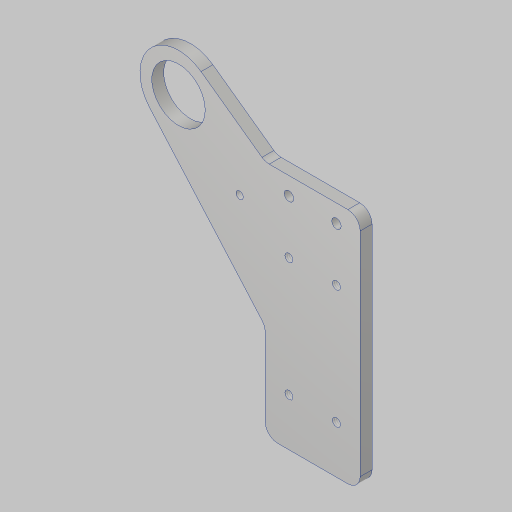
# Autodesk Inventor part: CL7-GB-008
Saved by Autodesk Inventor 2023.5 (Build 275446000, 446)
## iProperties
Created: 2025-03-18
Part Number: CL7-GB-008
Material: Aluminum 6061
Document SubType Name: Modeling
Designer: slick
Density: 2.7 g/cm^3
Appearance: Aluminum - Flat
Mass: 158.098 g
Surface Area: 311.728 cm^2
Volume: 58.555 cm^3
Author: slick
Autodesk Inventor part; units mm, degrees
ref_plane "YZ Plane" through (0, 0, 0) normal (1, 0, 0) x (0, 1, 0)
ref_plane "XZ Plane" through (0, 0, 0) normal (0, 1, 0) x (-1, 0, 0)
ref_plane "XY Plane" through (0, 0, 0) normal (0, 0, 1) x (1, 0, 0)
sketch "Sketch1" plane through (0, 0, 0) normal (0, 0, 1) x (1, 0, 0)
  line L0 (0, 0) -> (-50.8, 0) construction
  line L1 (-50.8, 0) -> (-50.8, 381) construction
  line L2 (-50.8, 381) -> (0, 381) construction
  line L3 (0, 381) -> (0, 0) construction
  circle A0 centre (-50.8, 431.8) radius 11.1125 construction
  line L4 (-50.8, 353.7099) -> (-298.4703, 0) construction
  line L5 (-298.4703, 0) -> (-267.4626, 0) construction
  line L6 (-267.4626, 0) -> (-50.8, 309.4263) construction
  dimension "d0" = 50.8
  dimension "d1" = 381
  dimension "d2" = 22.225
  dimension "d3" = 431.8
  dimension "d4" = 50.8
  dimension "d5" = 431.8
  dimension "d6" = 25.4
  dimension "d7" = 35
  constraints: 14 end point, 3 parallel, 2 horizontal, 2 point on line, 1 centre point, 1 collinear, 1 perpendicular
  measures "d0" distance of L1.end L2.end
  measures "d1" distance of L0.end L1.end
  measures "d2" diameter of A0
  measures "d3" distance from line of L0 A0.centre
  measures "d4" distance from line of L3 A0.centre
  measures "d5" distance of L4.start L4.end
  measures "d6" distance between parallel lines of L6 L4
  measures "d7" angle of L1 L4
sketch "Sketch2" plane through (0, 0, 0) normal (0, 0, 1) x (1, 0, 0)
  line L0 (-267.4626, 0) -> (-50.8, 309.4263) construction
  line L1 (-50.8, 353.7099) -> (-298.4703, 0) construction
  line L2 (-50.8, 0) -> (-50.8, 381) construction
  line L3 (0, 381) -> (0, 0) construction
  line L4 (-50.8, 381) -> (0, 381) construction
  circle A0 centre (-50.8, 431.8) radius 11.1125 construction
  line L5 (0, 0) -> (-50.8, 0) construction
  line L6 (-298.4703, 0) -> (-267.4626, 0) construction
  circle A1 centre (-88.9, 38.1) radius 30.48 construction
  circle A2 centre (-88.9, 38.1) radius 6.35 construction
  circle A3 centre (-124.3919, 76.2) radius 45.72 construction
  circle A4 centre (-124.3919, 76.2) radius 11.43 construction
  circle A5 centre (-101.6, 129.9906) radius 46.99 construction
  circle A6 centre (-101.6, 129.9906) radius 12.7 construction
  circle A7 centre (-97.155, 185.6935) radius 43.18 construction
  circle A8 centre (-124.3919, 76.2) radius 14.2875
  circle A9 centre (-101.6, 129.9906) radius 14.2875
  circle A10 centre (-97.155, 185.6935) radius 14.2875
  circle A11 centre (-50.8, 431.8) radius 54.5719 construction
  line L7 (-50.8, 177.8) -> (0, 177.8)
  circle A12 centre (-97.155, 185.6935) radius 20.6375 construction
  circle A13 centre (-101.6, 129.9906) radius 20.6375 construction
  circle A14 centre (-124.3919, 76.2) radius 20.6375 construction
  circle A15 centre (-88.9, 38.1) radius 25.4 construction
  line L8 (-50.8, 177.8) -> (-85.1131, 202.4536)
  line L9 (-141.8793, 65.2411) -> (-114.7275, 21.9145)
  line L10 (-74.6041, 11.1805) -> (0, 50.8)
  line L11 (0, 177.8) -> (0, 50.8)
  arc A16 (-141.8226, 87.2489) -> (-117.7308, 184.0988) centre (-275.3417, 171.8837) ccw
  arc A17 (-85.1131, 202.4536) -> (-117.7308, 184.0988) centre (-97.155, 185.6935) ccw
  arc A18 (-141.8226, 87.2489) -> (-141.8793, 65.2411) centre (-124.3919, 76.2) ccw
  arc A19 (-114.7275, 21.9145) -> (-74.6041, 11.1805) centre (-88.9, 38.1) ccw
  line L12 (-38.1, 152.4) -> (-38.1, 127) construction
  line L13 (-40.6527, 152.4) -> (-40.6527, 127)
  line L14 (-35.5473, 127) -> (-35.5473, 152.4)
  arc A20 (-35.5473, 152.4) -> (-40.6527, 152.4) centre (-38.1, 152.4) ccw
  arc A21 (-40.6527, 127) -> (-35.5473, 127) centre (-38.1, 127) ccw
  line L15 (-12.7, 152.4) -> (-12.7, 127) construction
  line L16 (-15.2527, 152.4) -> (-15.2527, 127)
  line L17 (-10.1473, 127) -> (-10.1473, 152.4)
  arc A22 (-10.1473, 152.4) -> (-15.2527, 152.4) centre (-12.7, 152.4) ccw
  arc A23 (-15.2527, 127) -> (-10.1473, 127) centre (-12.7, 127) ccw
  line L18 (-38.1, 139.7) -> (-12.7, 139.7) construction
  line L19 (-38.1, 88.9) -> (-38.1, 63.5) construction
  line L20 (-40.6527, 88.9) -> (-40.6527, 63.5)
  line L21 (-35.5473, 63.5) -> (-35.5473, 88.9)
  arc A24 (-35.5473, 88.9) -> (-40.6527, 88.9) centre (-38.1, 88.9) ccw
  arc A25 (-40.6527, 63.5) -> (-35.5473, 63.5) centre (-38.1, 63.5) ccw
  line L22 (-12.7, 88.9) -> (-12.7, 63.5) construction
  line L23 (-15.2527, 88.9) -> (-15.2527, 63.5)
  line L24 (-10.1473, 63.5) -> (-10.1473, 88.9)
  arc A26 (-10.1473, 88.9) -> (-15.2527, 88.9) centre (-12.7, 88.9) ccw
  arc A27 (-15.2527, 63.5) -> (-10.1473, 63.5) centre (-12.7, 63.5) ccw
  line L25 (-38.1, 76.2) -> (-12.7, 76.2) construction
  circle A28 centre (-88.9, 38.1) radius 10.795
  line L26 (-112.6649, 172.0793) -> (-50.8, 101.6)
  line L27 (-50.8, 101.6) -> (-50.8, 23.822)
  arc A29 (-117.7308, 184.0988) -> (-112.6649, 172.0793) centre (-97.155, 185.6935) ccw
  line L28 (0, 50.8) -> (-50.8, 50.8)
  point P0 (-88.9, 63.5)
  point P1 (-110.897, 50.8)
  point P2 (-110.897, 25.4)
  point P3 (-88.9, 12.7)
  point P4 (-66.903, 25.4)
  point P5 (-66.903, 50.8)
  point P6 (-25.4, 139.7)
  point P7 (-25.4, 177.8)
  point P8 (-25.4, 76.2)
  point P9 (-38.1, 168.275)
  point P10 (-12.7, 168.275)
  dimension "d25" = 50.8
  dimension "d8" = 60.96
  dimension "d9" = 12.7
  dimension "d10" = 91.44
  dimension "d11" = 38.1
  dimension "d12" = 38.1
  dimension "d13" = 22.86
  dimension "d14" = 93.98
  dimension "d15" = 25.4
  dimension "d16" = 86.36
  dimension "d17" = 76.2
  dimension "d20" = 50.8
  dimension "d22" = 28.575
  dimension "d23" = 109.1438
  dimension "d24" = 6.35
  dimension "d28" = 360
  dimension "d30" = 177.8
  dimension "d31" = 50.8
  dimension "d32" = 5.1054
  dimension "d33" = 25.4
  dimension "d34" = 38.1
  dimension "d35" = 25.4
  dimension "d36" = 5.1054
  dimension "d37" = 25.4
  dimension "d38" = 25.4
  dimension "d39" = 63.5
  dimension "d42" = 21.59
  dimension "d50" = 9.525
  dimension "d59" = 46.355
  dimension "d87" = 76.2
  constraints: 52 end point, 33 point on circle, 28 centre point, 27 tangent, 15 coincident, 7 midpoint, 7 point on line, 6 equal radius, 6 parallel, 6 vertical alignment, 5 horizontal alignment, 3 horizontal, 2 vertical, 1 collinear, 1 perpendicular, 9 other
  measures "d8" diameter of A1
  measures "d9" diameter of A2
  measures "d10" diameter of A3
  measures "d11" distance from line of L5 A1.centre
  measures "d12" distance from line of L2 A1.centre
  measures "d13" diameter of A4
  measures "d14" diameter of A5
  measures "d15" diameter of A6
  measures "d16" diameter of A7
  measures "d17" distance from line of L5 A3.centre
  measures "d20" distance from line of L2 A5.centre
  measures "d22" diameter of A8
  measures "d23" diameter of A11
  measures "d24" radial gap between concentric circles of A10 A12
  measures "d30" distance between parallel lines of L5 L7
  measures "d31" distance from line of L5 L10.end
  measures "d32" diameter of A21
  measures "d33" distance of L12.start L12.end
  measures "d34" distance from line of L7 L18.start
  measures "d35" distance of L18.start L18.end
  measures "d36" diameter of A25
  measures "d37" distance of L19.start L19.end
  measures "d38" distance of L25.start L25.end
  measures "d39" distance between parallel lines of L18 L25
  measures "d42" diameter of A28
  measures "d50" distance from line of L7 point (-38.1, 168.275)
  measures "d59" distance from line of L2 A7.centre
  measures "d87" distance from line of L7 L26.end
extrude "Extrusion1" add sketch "Sketch2" along normal blind 6.35 contours L7 L11 L28 L27 L26 A29 A17 L8 | A20 L14 A21 L13 | A22 L17 A23 L16 | A24 L21 A25 L20 | A26 L24 A27 L23
hole "Hole1" at (-88.9, 63.5, 0) at (-110.897, 50.8, 0) at (-110.897, 25.4, 0) at (-88.9, 12.7, 0) at (-66.903, 25.4, 0) at (-66.903, 50.8, 0) at (-38.1, 168.275, 0) at (-12.7, 168.275, 0) direction (0, 0, 1) diameter 5.1054 end through all clearance for "Flat Head Machine Screw (82)" size "#10" standard "Ansi Unified Screw Threads"
hole "Hole2" at (-12.7, 139.7, 0) at (-38.1, 139.7, 0) at (-38.1, 76.2, 0) at (-12.7, 76.2, 0) direction (0, 0, 1) diameter 4.3434 end through all thread size "12-24 UNC" class "2B" standard "ANSI Unified Screw Threads"
fillet "Fillet1" radius 6.604 3 edges at (-50.8, 177.8, 3.175) (0, 177.8, 3.175) (0, 50.8, 3.175)
sketch "Sketch4" plane through (0, 0, 6.35) normal (0, 0, 1) x (1, 0, 0)
  arc A0 (-6.604, 50.8) -> (0, 57.404) centre (-6.604, 57.404) ccw construction
  line L0 (0, 57.404) -> (0, 171.196) construction
  arc A1 (0, 171.196) -> (-6.604, 177.8) centre (-6.604, 171.196) ccw construction
  line L1 (-6.604, 177.8) -> (-48.6735, 177.8) construction
  arc A2 (-52.5269, 179.0408) -> (-48.6735, 177.8) centre (-48.6735, 184.404) ccw construction
  line L2 (-52.5269, 179.0408) -> (-85.1131, 202.4536) construction
  arc A3 (-85.1131, 202.4536) -> (-112.6649, 172.0793) centre (-97.155, 185.6935) ccw construction
  circle A4 centre (-38.1, 76.2) radius 2.1717 construction
  circle A5 centre (-12.7, 139.7) radius 2.1717 construction
  circle A6 centre (-38.1, 139.7) radius 2.1717 construction
  circle A7 centre (-12.7, 76.2) radius 2.1717 construction
  circle A8 centre (-38.1, 168.275) radius 2.5527 construction
  circle A9 centre (-12.7, 168.275) radius 2.5527 construction
  circle A10 centre (-97.155, 185.6935) radius 14.2875 construction
  line L3 (-112.6649, 172.0793) -> (-50.8, 101.6) projected
  line L4 (-50.8, 101.6) -> (-50.8, 50.8) projected
  line L5 (-50.8, 50.8) -> (-6.604, 50.8) projected
  point P0 (0, 0)
  point P1 (-64.4644, 155.575)
  dimension "d74" = 44.45
  dimension "d75" = 22.225
  measures "d74" distance of point (-64.464, 155.575) A3.centre
  measures "d75" distance from line of point (-64.464, 155.575) L1
hole "Hole3" at (-64.4644, 155.575, 6.35) direction (0, 0, -1) diameter 3.9624 end through all thread size "10-32 UNF" class "2B" standard "ANSI Unified Screw Threads"
fillet "Fillet3" radius 6.604 2 edges at (-50.8, 50.8, 3.175) (-50.8, 101.6, 3.175)
sketch "Sketch3" plane through (0, 0, 6.35) normal (0, 0, 1) x (1, 0, 0)
  arc A0 (-3.5066, 48.9378) -> (0, 54.7703) centre (-6.604, 54.7703) ccw construction
  line L0 (0, 54.7703) -> (0, 171.196) construction
  arc A1 (0, 171.196) -> (-6.604, 177.8) centre (-6.604, 171.196) ccw construction
  line L1 (-6.604, 177.8) -> (-48.6735, 177.8) construction
  arc A2 (-52.5269, 179.0408) -> (-48.6735, 177.8) centre (-48.6735, 184.404) ccw construction
  line L2 (-52.5269, 179.0408) -> (-85.1131, 202.4536) construction
  arc A3 (-85.1131, 202.4536) -> (-112.6649, 172.0793) centre (-97.155, 185.6935) ccw construction
  line L3 (-50.8, 23.822) -> (-3.5066, 48.9378) construction
  circle A4 centre (-38.1, 76.2) radius 2.1717 construction
  circle A5 centre (-12.7, 139.7) radius 2.1717 construction
  circle A6 centre (-38.1, 139.7) radius 2.1717 construction
  circle A7 centre (-12.7, 76.2) radius 2.1717 construction
  circle A8 centre (-38.1, 168.275) radius 2.5527 construction
  circle A9 centre (-12.7, 168.275) radius 2.5527 construction
  circle A10 centre (-97.155, 185.6935) radius 14.2875 construction
  arc A11 (-88.8183, 197.2966) -> (-111.3998, 184.5895) centre (-97.155, 185.6935) ccw construction
  line L4 (-88.8183, 197.2966) -> (-56.2321, 173.8838) construction
  arc A12 (-56.2321, 173.8838) -> (-48.6735, 171.45) centre (-48.6735, 184.404) ccw construction
  line L5 (-48.6735, 171.45) -> (-6.604, 171.45) construction
  arc A13 (-6.35, 171.196) -> (-6.604, 171.45) centre (-6.604, 171.196) ccw construction
  line L6 (-6.35, 171.196) -> (-6.35, 54.7703) construction
  arc A14 (-6.4849, 54.546) -> (-6.35, 54.7703) centre (-6.604, 54.7703) ccw
  line L7 (-6.4849, 54.546) -> (-77.5824, 16.7888) construction
  arc A15 (-109.3468, 25.2865) -> (-77.5824, 16.7888) centre (-88.9, 38.1) ccw construction
  line L8 (-109.3468, 25.2865) -> (-136.4985, 68.613) construction
  arc A16 (-136.4593, 83.8492) -> (-136.4985, 68.613) centre (-124.3919, 76.2) ccw construction
  arc A17 (-136.4593, 83.8492) -> (-111.3998, 184.5895) centre (-275.3417, 171.8837) ccw construction
  circle A18 centre (-97.155, 185.6935) radius 20.6375 construction
  circle A19 centre (-38.1, 168.275) radius 8.9027 construction
  circle A20 centre (-101.6, 129.9906) radius 20.6375 construction
  circle A21 centre (-124.3919, 76.2) radius 20.6375 construction
  circle A22 centre (-88.9, 63.5) radius 2.5527 construction
  circle A23 centre (-88.9, 63.5) radius 8.9027 construction
  circle A24 centre (-66.903, 50.8) radius 8.9027 construction
  circle A25 centre (-38.1, 76.2) radius 8.9027 construction
  circle A26 centre (-12.7, 76.2) radius 2.1717 construction
  circle A27 centre (-12.7, 76.2) radius 8.9027 construction
  circle A28 centre (-38.1, 139.7) radius 8.9027 construction
  circle A29 centre (-12.7, 139.7) radius 2.1717 construction
  circle A30 centre (-12.7, 139.7) radius 8.9027 construction
  circle A31 centre (-12.7, 168.275) radius 2.5527 construction
  circle A32 centre (-12.7, 168.275) radius 8.9027 construction
  circle A33 centre (-38.1, 139.7) radius 2.1717 construction
  line L9 (-101.6, 129.9906) -> (-38.1, 139.7) construction
  circle A34 centre (-38.1, 76.2) radius 2.1717 construction
  line L10 (-38.1, 139.7) -> (-38.1, 76.2) construction
  line L11 (-38.1, 76.2) -> (-66.903, 50.8) construction
  line L12 (-66.903, 50.8) -> (-88.9, 63.5) construction
  line L13 (-88.9, 63.5) -> (-124.3919, 76.2) construction
  circle A35 centre (-38.1, 168.275) radius 2.5527 construction
  line L14 (-38.1, 139.7) -> (-38.1, 168.275) construction
  line L15 (-38.1, 107.95) -> (-6.35, 107.95) construction
  line L16 (-55.1495, 28.702) -> (-62.7133, 42.9448) construction
  line L17 (-101.1201, 126.852) -> (-41.275, 136.0026) construction
  line L18 (-41.275, 136.0026) -> (-41.275, 77.6333) construction
  line L19 (-41.275, 77.6333) -> (-67.2915, 54.6905) construction
  line L20 (-67.2915, 54.6905) -> (-87.5606, 66.3929) construction
  line L21 (-87.5606, 66.3929) -> (-123.3222, 79.1894) construction
  line L22 (-102.0799, 133.1291) -> (-34.925, 143.3974) construction
  line L23 (-34.925, 143.3974) -> (-34.925, 74.7667) construction
  line L24 (-34.925, 74.7667) -> (-66.5144, 46.9095) construction
  line L25 (-66.5144, 46.9095) -> (-90.2394, 60.6071) construction
  line L26 (-90.2394, 60.6071) -> (-125.4616, 73.2106) construction
  line L27 (-34.925, 139.7) -> (-34.925, 168.275) construction
  line L28 (-41.275, 139.7) -> (-41.275, 168.275) construction
  line L29 (-38.1, 111.125) -> (-6.35, 111.125) construction
  line L30 (-38.1, 104.775) -> (-6.35, 104.775) construction
  line L31 (-76.7242, 188.6072) -> (-56.2321, 173.8838)
  line L32 (-48.6735, 171.45) -> (-46.4173, 171.45)
  line L33 (-29.7827, 171.45) -> (-21.0173, 171.45)
  line L34 (-6.35, 162.0352) -> (-6.35, 145.9398)
  line L35 (-34.925, 159.9577) -> (-34.925, 148.0173)
  line L36 (-41.275, 159.9577) -> (-41.275, 148.0173)
  line L37 (-34.925, 131.3827) -> (-34.925, 84.5173)
  line L38 (-41.275, 131.3827) -> (-41.275, 84.5173)
  line L39 (-6.35, 133.4602) -> (-6.35, 82.4398)
  line L40 (-6.35, 69.9602) -> (-6.35, 54.7703)
  line L41 (-6.4849, 54.546) -> (-55.1495, 28.702)
  line L42 (-55.1495, 28.702) -> (-62.7133, 42.9448)
  line L43 (-58.5648, 53.9198) -> (-42.2382, 68.3175)
  line L44 (-46.4381, 73.0802) -> (-62.7648, 58.6825)
  line L45 (-72.5184, 57.7083) -> (-80.1095, 62.091)
  line L46 (-95.6614, 69.2915) -> (-104.1226, 72.3192)
  line L47 (-45.8418, 135.3043) -> (-80.9626, 129.9342)
  line L48 (-46.8016, 141.5814) -> (-81.9224, 136.2113)
  line L49 (-6.35, 111.125) -> (-34.925, 111.125)
  line L50 (-34.925, 104.775) -> (-6.35, 104.775)
  arc A36 (-110.9157, 170.3133) -> (-76.7242, 188.6072) centre (-97.155, 185.6935) ccw
  arc A37 (-81.9224, 136.2113) -> (-112.7474, 147.3584) centre (-101.6, 129.9906) ccw
  arc A38 (-119.4378, 119.6117) -> (-80.9626, 129.9342) centre (-101.6, 129.9906) ccw
  arc A39 (-104.1226, 72.3192) -> (-129.3429, 96.2348) centre (-124.3919, 76.2) ccw
  arc A40 (-80.1095, 62.091) -> (-95.6614, 69.2915) centre (-88.9, 63.5) ccw
  arc A41 (-62.7648, 58.6825) -> (-72.5184, 57.7083) centre (-66.903, 50.8) ccw
  arc A42 (-62.7133, 42.9448) -> (-58.5648, 53.9198) centre (-66.903, 50.8) ccw
  arc A43 (-41.275, 84.5173) -> (-46.4381, 73.0802) centre (-38.1, 76.2) ccw
  arc A44 (-42.2382, 68.3175) -> (-34.925, 84.5173) centre (-38.1, 76.2) ccw
  arc A45 (-6.35, 82.4398) -> (-6.35, 69.9602) centre (-12.7, 76.2) ccw
  arc A46 (-45.8418, 135.3043) -> (-41.275, 131.3827) centre (-38.1, 139.7) ccw
  arc A47 (-6.35, 145.9398) -> (-6.35, 133.4602) centre (-12.7, 139.7) ccw
  arc A48 (-41.275, 148.0173) -> (-46.8016, 141.5814) centre (-38.1, 139.7) ccw
  arc A49 (-34.925, 131.3827) -> (-34.925, 148.0173) centre (-38.1, 139.7) ccw
  arc A50 (-46.4173, 171.45) -> (-41.275, 159.9577) centre (-38.1, 168.275) ccw
  arc A51 (-34.925, 159.9577) -> (-29.7827, 171.45) centre (-38.1, 168.275) ccw
  arc A52 (-21.0173, 171.45) -> (-6.35, 162.0352) centre (-12.7, 168.275) ccw
  arc A53 (-56.2321, 173.8838) -> (-48.6735, 171.45) centre (-48.6735, 184.404) ccw
  arc A54 (-112.7474, 147.3584) -> (-110.9157, 170.3133) centre (-275.3417, 171.8837) ccw
  arc A55 (-129.3429, 96.2348) -> (-119.4378, 119.6117) centre (-275.3417, 171.8837) ccw
  circle A56 centre (-64.4644, 155.575) radius 1.9812 construction
  circle A57 centre (-64.4644, 155.575) radius 1.9812 construction
  circle A58 centre (-64.4644, 155.575) radius 8.9027 construction
  line L51 (-97.155, 185.6935) -> (-64.4644, 155.575) construction
  line L52 (-64.4644, 155.575) -> (-38.1, 168.275) construction
  line L53 (-95.0037, 188.0285) -> (-63.8992, 159.3714) construction
  line L54 (-63.8992, 159.3714) -> (-39.4779, 171.1354) construction
  line L55 (-36.7221, 165.4146) -> (-65.0295, 151.7786) construction
  line L56 (-65.0295, 151.7786) -> (-99.3063, 183.3585) construction
  line L57 (-46.9711, 167.5259) -> (-58.349, 162.045)
  line L58 (-44.2153, 161.805) -> (-55.5932, 156.3241)
  line L59 (-72.7326, 158.8756) -> (-84.3092, 169.5413)
  line L60 (-80.0066, 174.2114) -> (-68.43, 163.5457)
  arc A59 (-58.349, 162.045) -> (-68.43, 163.5457) centre (-64.4644, 155.575) ccw
  arc A60 (-72.7326, 158.8756) -> (-55.5932, 156.3241) centre (-64.4644, 155.575) ccw
  line L61 (-112.6649, 172.0793) -> (-50.8, 101.6) projected
  line L62 (-50.8, 101.6) -> (-50.8, 23.822) projected
  point P0 (0, 0)
  point P1 (-6.35, 104.775)
  dimension "d61" = 6.35
  dimension "d62" = 6.35
  dimension "d63" = 25.4
  dimension "d64" = 3.175
  dimension "d65" = 3.175
  dimension "d66" = 3.175
  dimension "d67" = 3.175
  dimension "d68" = 3.175
  dimension "d69" = 3.175
  dimension "d83" = 3.175
  dimension "d84" = 3.175
  constraints: 112 end point, 102 point on circle, 40 centre point, 38 point on line, 29 coincident, 9 equal radius, 6 collinear, 4 parallel, 3 vertical, 1 horizontal, 1 midpoint, 1 perpendicular, 31 other
  measures "d61" radial gap between concentric circles of A10 A18
  measures "d62" radial gap between concentric circles of A8 A19
  measures "d63" distance from line of A15.centre L16
  measures "d64" distance between parallel lines of L9 L17
  measures "d65" distance between parallel lines of L9 L22
  measures "d66" distance between parallel lines of L14 L27
  measures "d67" distance between parallel lines of L14 L28
  measures "d68" distance between parallel lines of L15 L29
  measures "d69" distance between parallel lines of L15 L30
  measures "d83" distance between parallel lines of L51 L53
  measures "d84" distance between parallel lines of L52 L55
body "Solid1"
